Autodesk Fusion 360 part; units mm, degrees
(part 5 of 5)
component "TSSOP16_001" placed x (1, 0, 0) y (0, -1, 0) z (0, 0, -1) at (20.815, 10.6871, 0.1) in component "TSSOP16_010"
component "TSSOP16_002" placed x (1, 0, 0) y (0, -1, 0) z (0, 0, -1) at (20.815, 10.6871, 0.1) in component "TSSOP16_010"
component "TSSOP16_003" placed x (1, 0, 0) y (0, -1, 0) z (0, 0, -1) at (20.815, 10.6871, 0.1) in component "TSSOP16_010"
component "TSSOP16_004" placed x (1, 0, 0) y (0, -1, 0) z (0, 0, -1) at (20.815, 10.6871, 0.1) in component "TSSOP16_010"
component "TSSOP16_005" placed x (1, 0, 0) y (0, -1, 0) z (0, 0, -1) at (20.815, 10.6871, 0.1) in component "TSSOP16_010"
component "TSSOP16_006" placed x (1, 0, 0) y (0, -1, 0) z (0, 0, -1) at (20.815, 10.6871, 0.1) in component "TSSOP16_010"
component "TSSOP16_007" placed x (1, 0, 0) y (0, -1, 0) z (0, 0, -1) at (20.815, 10.6871, 0.1) in component "TSSOP16_010"
component "TSSOP16_008" placed x (1, 0, 0) y (0, -1, 0) z (0, 0, -1) at (20.815, 10.6871, 0.1) in component "TSSOP16_010"
component "TSSOP16_009" placed x (1, 0, 0) y (0, -1, 0) z (0, 0, -1) at (20.815, 10.6871, 0.1) in component "TSSOP16_010"
component "ShapeString253" placed x (1, 0, 0) y (0, 1, 0) z (0, 0, 1) at (0, 0, 0) in component "TSSOP16_010"
component "ShapeString001" placed x (1, 0, 0) y (0, 1, 0) z (0, 0, 1) at (-3.2, -0.84, 0) in component "ShapeString256"
component "ShapeString254" placed x (1, 0, 0) y (0, 1, 0) z (0, 0, 1) at (-3.2, -0.84, 0) in component "ShapeString256"
component "ShapeString255" placed x (1, 0, 0) y (0, 1, 0) z (0, 0, 1) at (-3.2, -0.84, 0) in component "ShapeString256"
component "ShapeString256" placed x (1, 0, 0) y (0, 1, 0) z (0, 0, 1) at (0, 0, 0) in component "Part010"
component "body" placed x (1, 0, 0) y (0, 1, 0) z (0, 0, 1) at (0, 0, 0) in component "SMD_resistor001"
component "contact1" placed x (1, 0, 0) y (0, 1, 0) z (0, 0, 1) at (0, -0.8, 0) in component "SMD_resistor001"
component "contact2" placed x (-1, 0, 0) y (0, -1, 0) z (0, 0, 1) at (0, 0.8, 0) in component "SMD_resistor001"
component "label" placed x (1, 0, 0) y (0, 1, 0) z (0, 0, 1) at (0, 0, 0.2) in component "SMD_resistor001"
component "Part010" placed x (0, 1, 0) y (-1, 0, 0) z (0, 0, 1) at (-0.66, 2.73, 0.24) in component "SMD_resistor001"
component "ShapeString002" placed x (1, 0, 0) y (0, 1, 0) z (0, 0, 1) at (-3.2, -0.84, 0) in component "ShapeString259"
component "ShapeString257" placed x (1, 0, 0) y (0, 1, 0) z (0, 0, 1) at (-3.2, -0.84, 0) in component "ShapeString259"
component "ShapeString258" placed x (1, 0, 0) y (0, 1, 0) z (0, 0, 1) at (-3.2, -0.84, 0) in component "ShapeString259"
component "ShapeString259" placed x (1, 0, 0) y (0, 1, 0) z (0, 0, 1) at (0, 0, 0) in component "Part013"
component "body003" placed x (1, 0, 0) y (0, 1, 0) z (0, 0, 1) at (0, 0, 0) in component "SMD_resistor002"
component "contact016" placed x (1, 0, 0) y (0, 1, 0) z (0, 0, 1) at (0, -0.8, 0) in component "SMD_resistor002"
component "contact017" placed x (-1, 0, 0) y (0, -1, 0) z (0, 0, 1) at (0, 0.8, 0) in component "SMD_resistor002"
component "label001" placed x (1, 0, 0) y (0, 1, 0) z (0, 0, 1) at (0, 0, 0.2) in component "SMD_resistor002"
component "Part013" placed x (0, 1, 0) y (-1, 0, 0) z (0, 0, 1) at (-0.66, 2.73, 0.24) in component "SMD_resistor002"
component "ShapeString003" placed x (1, 0, 0) y (0, 1, 0) z (0, 0, 1) at (-3.2, -0.84, 0) in component "ShapeString262"
component "ShapeString260" placed x (1, 0, 0) y (0, 1, 0) z (0, 0, 1) at (-3.2, -0.84, 0) in component "ShapeString262"
component "ShapeString261" placed x (1, 0, 0) y (0, 1, 0) z (0, 0, 1) at (-3.2, -0.84, 0) in component "ShapeString262"
component "ShapeString262" placed x (1, 0, 0) y (0, 1, 0) z (0, 0, 1) at (0, 0, 0) in component "Part015"
component "body004" placed x (1, 0, 0) y (0, 1, 0) z (0, 0, 1) at (0, 0, 0) in component "SMD_resistor003"
component "contact018" placed x (1, 0, 0) y (0, 1, 0) z (0, 0, 1) at (0, -0.8, 0) in component "SMD_resistor003"
component "contact019" placed x (-1, 0, 0) y (0, -1, 0) z (0, 0, 1) at (0, 0.8, 0) in component "SMD_resistor003"
component "label002" placed x (1, 0, 0) y (0, 1, 0) z (0, 0, 1) at (0, 0, 0.2) in component "SMD_resistor003"
component "Part015" placed x (0, 1, 0) y (-1, 0, 0) z (0, 0, 1) at (-0.66, 2.73, 0.24) in component "SMD_resistor003"
component "ShapeString004" placed x (1, 0, 0) y (0, 1, 0) z (0, 0, 1) at (-3.2, -0.84, 0) in component "ShapeString265"
component "ShapeString263" placed x (1, 0, 0) y (0, 1, 0) z (0, 0, 1) at (-3.2, -0.84, 0) in component "ShapeString265"
component "ShapeString264" placed x (1, 0, 0) y (0, 1, 0) z (0, 0, 1) at (-3.2, -0.84, 0) in component "ShapeString265"
component "ShapeString265" placed x (1, 0, 0) y (0, 1, 0) z (0, 0, 1) at (0, 0, 0) in component "Part017"
component "body005" placed x (1, 0, 0) y (0, 1, 0) z (0, 0, 1) at (0, 0, 0) in component "SMD_resistor004"
component "contact020" placed x (1, 0, 0) y (0, 1, 0) z (0, 0, 1) at (0, -0.8, 0) in component "SMD_resistor004"
component "contact021" placed x (-1, 0, 0) y (0, -1, 0) z (0, 0, 1) at (0, 0.8, 0) in component "SMD_resistor004"
component "label003" placed x (1, 0, 0) y (0, 1, 0) z (0, 0, 1) at (0, 0, 0.2) in component "SMD_resistor004"
component "Part017" placed x (0, 1, 0) y (-1, 0, 0) z (0, 0, 1) at (-0.66, 2.73, 0.24) in component "SMD_resistor004"
component "ShapeString005" placed x (1, 0, 0) y (0, 1, 0) z (0, 0, 1) at (-3.2, -0.84, 0) in component "ShapeString268"
component "ShapeString266" placed x (1, 0, 0) y (0, 1, 0) z (0, 0, 1) at (-3.2, -0.84, 0) in component "ShapeString268"
component "ShapeString267" placed x (1, 0, 0) y (0, 1, 0) z (0, 0, 1) at (-3.2, -0.84, 0) in component "ShapeString268"
component "ShapeString268" placed x (1, 0, 0) y (0, 1, 0) z (0, 0, 1) at (0, 0, 0) in component "Part019"
component "body006" placed x (1, 0, 0) y (0, 1, 0) z (0, 0, 1) at (0, 0, 0) in component "SMD_resistor005"
component "contact022" placed x (1, 0, 0) y (0, 1, 0) z (0, 0, 1) at (0, -0.8, 0) in component "SMD_resistor005"
component "contact023" placed x (-1, 0, 0) y (0, -1, 0) z (0, 0, 1) at (0, 0.8, 0) in component "SMD_resistor005"
component "label004" placed x (1, 0, 0) y (0, 1, 0) z (0, 0, 1) at (0, 0, 0.2) in component "SMD_resistor005"
component "Part019" placed x (0, 1, 0) y (-1, 0, 0) z (0, 0, 1) at (-0.66, 2.73, 0.24) in component "SMD_resistor005"
component "ShapeString006" placed x (1, 0, 0) y (0, 1, 0) z (0, 0, 1) at (-3.2, -0.84, 0) in component "ShapeString271"
component "ShapeString269" placed x (1, 0, 0) y (0, 1, 0) z (0, 0, 1) at (-3.2, -0.84, 0) in component "ShapeString271"
component "ShapeString270" placed x (1, 0, 0) y (0, 1, 0) z (0, 0, 1) at (-3.2, -0.84, 0) in component "ShapeString271"
component "ShapeString271" placed x (1, 0, 0) y (0, 1, 0) z (0, 0, 1) at (0, 0, 0) in component "Part021"
component "body007" placed x (1, 0, 0) y (0, 1, 0) z (0, 0, 1) at (0, 0, 0) in component "SMD_resistor006"
component "contact024" placed x (1, 0, 0) y (0, 1, 0) z (0, 0, 1) at (0, -0.8, 0) in component "SMD_resistor006"
component "contact025" placed x (-1, 0, 0) y (0, -1, 0) z (0, 0, 1) at (0, 0.8, 0) in component "SMD_resistor006"
component "label005" placed x (1, 0, 0) y (0, 1, 0) z (0, 0, 1) at (0, 0, 0.2) in component "SMD_resistor006"
component "Part021" placed x (0, 1, 0) y (-1, 0, 0) z (0, 0, 1) at (-0.66, 2.73, 0.24) in component "SMD_resistor006"
component "body008" placed x (1, 0, 0) y (0, 1, 0) z (0, 0, 1) at (0, 0, -0.015) in component "SMD_cap001"
component "contact026" placed x (1, 0, 0) y (0, 1, 0) z (0, 0, 1) at (0, 0.95, 0) in component "SMD_cap001"
component "contact027" placed x (-1, 0, 0) y (0, -1, 0) z (0, 0, 1) at (0, -0.94, 0) in component "SMD_cap001"
component "body002" placed x (1, 0, 0) y (0, 1, 0) z (0, 0, 1) at (0, 0, -0.015) in component "SMD_cap002"
component "contact014" placed x (1, 0, 0) y (0, 1, 0) z (0, 0, 1) at (0, 0.95, 0) in component "SMD_cap002"
component "contact015" placed x (-1, 0, 0) y (0, -1, 0) z (0, 0, 1) at (0, -0.94, 0) in component "SMD_cap002"
component "ShapeString064" placed x (1, 0, 0) y (0, 1, 0) z (0, 0, 1) at (-0.88, -0.26, 0.72) in component "ShapeString274"
component "ShapeString272" placed x (1, 0, 0) y (0, 1, 0) z (0, 0, 1) at (-0.88, -0.26, 0.72) in component "ShapeString274"
component "ShapeString273" placed x (1, 0, 0) y (0, 1, 0) z (0, 0, 1) at (-0.88, -0.26, 0.72) in component "ShapeString274"
component "ShapeString274" placed x (1, 0, 0) y (0, 1, 0) z (0, 0, 1) at (0, 0, 0) in component "SOT23"
component "Pin036" placed x (-1, 0, 0) y (0, -1, 0) z (0, 0, 1) at (0.905, -0.235, 0) in component "SOT23"
component "Pin035" placed x (-1, 0, 0) y (0, -1, 0) z (0, 0, 1) at (-0.965, -0.215, 0) in component "SOT23"
component "Pin1" placed x (1, 0, 0) y (0, 1, 0) z (0, 0, 1) at (0, 0.295, 0) in component "SOT23"
component "Case" placed x (1, 0, 0) y (0, 1, 0) z (0, 0, 1) at (0, 0, 0) in component "SOT23"
component "ShapeString065" placed x (1, 0, 0) y (0, 1, 0) z (0, 0, 1) at (-0.98, -0.36, 0.72) in component "ShapeString278"
component "ShapeString275" placed x (1, 0, 0) y (0, 1, 0) z (0, 0, 1) at (-0.98, -0.36, 0.72) in component "ShapeString278"
component "ShapeString276" placed x (1, 0, 0) y (0, 1, 0) z (0, 0, 1) at (-0.98, -0.36, 0.72) in component "ShapeString278"
component "ShapeString277" placed x (1, 0, 0) y (0, 1, 0) z (0, 0, 1) at (-0.98, -0.36, 0.72) in component "ShapeString278"
component "ShapeString278" placed x (1, 0, 0) y (0, 1, 0) z (0, 0, 1) at (0, 0, 0) in component "SOT23-1"
component "Pin039" placed x (-1, 0, 0) y (0, -1, 0) z (0, 0, 1) at (0.905, -0.235, 0) in component "SOT23-1"
component "Pin038" placed x (-1, 0, 0) y (0, -1, 0) z (0, 0, 1) at (-0.965, -0.215, 0) in component "SOT23-1"
component "Pin037" placed x (1, 0, 0) y (0, 1, 0) z (0, 0, 1) at (0, 0.295, 0) in component "SOT23-1"
component "Case001" placed x (1, 0, 0) y (0, 1, 0) z (0, 0, 1) at (0, 0, 0) in component "SOT23-1"
component "TSSOP16_010" placed x (0, -1, 0) y (1, 0, 0) z (0, 0, 1) at (-0.13, 1.12, -1.67) in component "parts"
component "SMD_resistor001" placed x (0, -1, 0) y (-1, 0, 0) z (0, 0, -1) at (-4.35, -27.4, -1.61) in component "parts"
component "SMD_resistor002" placed x (0, -1, 0) y (-1, 0, 0) z (0, 0, -1) at (-4.35, -20.25, -1.61) in component "parts"
component "SMD_resistor003" placed x (0, -1, 0) y (-1, 0, 0) z (0, 0, -1) at (13.1, -26.91, -1.61) in component "parts"
component "SMD_resistor004" placed x (0, -1, 0) y (-1, 0, 0) z (0, 0, -1) at (2.65, 0.38, -1.61) in component "parts"
component "SMD_resistor005" placed x (0, -1, 0) y (-1, 0, 0) z (0, 0, -1) at (2.65, 2.72, -1.61) in component "parts"
component "SMD_resistor006" placed x (0, -1, 0) y (-1, 0, 0) z (0, 0, -1) at (2.65, 4.99, -1.61) in component "parts"
component "SMD_cap001" placed x (0, -1, 0) y (1, 0, 0) z (0, 0, 1) at (13.15, -25.1, -2.1) in component "parts"
component "SMD_cap002" placed x (0, -1, 0) y (1, 0, 0) z (0, 0, 1) at (3, -20.2, -2.1) in component "parts"
component "SOT23" placed x (1, 0, 0) y (0, -1, 0) z (0, 0, -1) at (-4.1, -23.68, -2.02) in component "parts"
component "SOT23-1" placed x (0, -1, 0) y (-1, 0, 0) z (0, 0, -1) at (2.67, -24, -2.02) in component "parts"
component "Frame" placed x (1, 0, 0) y (0, 1, 0) z (0, 0, 1) at (0, 0, 2.5) in component "pls-14"
component "Pin01" placed x (1, 0, 0) y (0, 1, 0) z (0, 0, 1) at (-16.51, 0, 0) in component "pls-14"
component "Pin002" placed x (1, 0, 0) y (0, 1, 0) z (0, 0, 1) at (-13.97, 0, 0) in component "pls-14"
component "Pin003" placed x (1, 0, 0) y (0, 1, 0) z (0, 0, 1) at (-11.43, 0, 0) in component "pls-14"
component "Pin004" placed x (1, 0, 0) y (0, 1, 0) z (0, 0, 1) at (-8.89, 0, 0) in component "pls-14"
component "Pin005" placed x (1, 0, 0) y (0, 1, 0) z (0, 0, 1) at (-6.35, 0, 0) in component "pls-14"
component "Pin006" placed x (1, 0, 0) y (0, 1, 0) z (0, 0, 1) at (-3.81, 0, 0) in component "pls-14"
component "Pin007" placed x (1, 0, 0) y (0, 1, 0) z (0, 0, 1) at (-1.27, 0, 0) in component "pls-14"
component "Pin008" placed x (1, 0, 0) y (0, 1, 0) z (0, 0, 1) at (1.27, 0, 0) in component "pls-14"
component "Pin009" placed x (1, 0, 0) y (0, 1, 0) z (0, 0, 1) at (3.81, 0, 0) in component "pls-14"
component "Pin010" placed x (1, 0, 0) y (0, 1, 0) z (0, 0, 1) at (6.35, 0, 0) in component "pls-14"
component "Pin011" placed x (1, 0, 0) y (0, 1, 0) z (0, 0, 1) at (8.89, 0, 0) in component "pls-14"
component "Pin012" placed x (1, 0, 0) y (0, 1, 0) z (0, 0, 1) at (11.43, 0, 0) in component "pls-14"
component "Pin013" placed x (1, 0, 0) y (0, 1, 0) z (0, 0, 1) at (13.97, 0, 0) in component "pls-14"
component "Pin014" placed x (1, 0, 0) y (0, 1, 0) z (0, 0, 1) at (16.51, 0, 0) in component "pls-14"
component "SD slot" placed x (0, 1, 0) y (1, 0, 0) z (0, 0, -1) at (-16.32, 3.6, -0.3) in component "components"
component "parts" placed x (1, 0, 0) y (0, 1, 0) z (0, 0, 1) at (0, 0, 1.31) in component "components"
component "pls-14" placed x (-1, 0, 0) y (0, 1, 0) z (0, 0, -1) at (0, -41, 2.28) in component "components"
component "plate and holes" placed x (1, 0, 0) y (0, 1, 0) z (0, 0, 1) at (0, 0, 0) in component "Board"
component "silk_upper" placed x (1, 0, 0) y (0, 1, 0) z (0, 0, 1) at (0, 0, 1.82) in component "Board"
component "cupper_upper" placed x (1, 0, 0) y (0, 1, 0) z (0, 0, 1) at (0, 0, 1.6) in component "Board"
component "cupper_bottom" placed x (1, 0, 0) y (0, 1, 0) z (0, 0, 1) at (0, 0, -0.1) in component "Board"
component "mask_bottom" placed x (1, 0, 0) y (0, 1, 0) z (0, 0, 1) at (0, 0, -0.2) in component "Board"
component "silk_bottom" placed x (1, 0, 0) y (0, 1, 0) z (0, 0, 1) at (0, 0, -0.01) in component "Board"
component "components" placed x (1, 0, 0) y (0, 1, 0) z (0, 0, 1) at (0, 0, 0) in component "Board"
component "mask_upper" placed x (1, 0, 0) y (0, 1, 0) z (0, 0, 1) at (0, 0, 1.7) in component "Board"
component "light_shelf" placed x (1, 0, 0) y (0, 0, -1) z (0, 1, 0) at (0, -30.43, -30.75) in component "tft_cable"
component "main_shelf" placed x (1, 0, 0) y (0, 1, 0) z (0, 0, 1) at (0, 0, 0) in component "tft_cable"
component "tft_cable" placed x (1, 0, 0) y (0, -1, 0) z (0, 0, -1) at (-12.5, -65.5, -0.43) in component "tft"
component "tft_matrix" placed x (1, 0, 0) y (0, 1, 0) z (0, 0, 1) at (0, 2.96, 1.5) in component "tft"
component "tft_board" placed x (1, 0, 0) y (0, 1, 0) z (0, 0, 1) at (0, 0, 0) in component "tft"
component "screen_film" placed x (1, 0, 0) y (0, 1, 0) z (0, 0, 1) at (0, 0, 0) in component "screen"
component "screen_glass" placed x (1, 0, 0) y (0, 1, 0) z (0, 0, 1) at (0, 0, 0.22) in component "screen"
component "frame" placed x (1, 0, 0) y (0, 1, 0) z (0, 0, 1) at (0, 2, 0.23) in component "Display"
component "metal bandage" placed x (1, 0, 0) y (0, 1, 0) z (0, 0, 1) at (0, 0, 0) in component "Display"
component "tft" placed x (1, 0, 0) y (0, 1, 0) z (0, 0, 1) at (0, 2.3, 0.65) in component "Display"
component "screen" placed x (1, 0, 0) y (0, 1, 0) z (0, 0, 1) at (0, 2, 2.65) in component "Display"
component "ShapeString068" placed x (0, 1, 0) y (1, 0, 0) z (0, 0, -1) at (16.1, -39.5, 0) in component "touch_cable"
component "touch_cable_contacts" placed x (1, 0, 0) y (0, 1, 0) z (0, 0, 1) at (0, 0, 0) in component "touch_cable"
component "touch_cable_film" placed x (1, 0, 0) y (0, 1, 0) z (0, 0, 1) at (0, 0, 0.1) in component "touch_cable"
component "touch_routs" placed x (1, 0, 0) y (0, 1, 0) z (0, 0, 1) at (0, 0, 0.05) in component "Touchscreen"
component "touch_protect" placed x (1, 0, 0) y (0, 1, 0) z (0, 0, 1) at (0, 0, 0.15) in component "Touchscreen"
component "touch_cable" placed x (1, 0, 0) y (0, 1, 0) z (0, 0, 1) at (-12.6, -4, 3.7) in component "Touchscreen"
component "Display" placed x (1, 0, 0) y (0, 1, 0) z (0, 0, 1) at (0, 0, 0) in component "Display and Touchscreen"
component "Touchscreen" placed x (1, 0, 0) y (0, 1, 0) z (0, 0, 1) at (0, 0, 0) in component "Display and Touchscreen"
component "Board" placed x (1, 0, 0) y (0, 1, 0) z (0, 0, 1) at (0, 0, 0) in component "2.8''LCD_MSP2807"
component "Display and Touchscreen" placed x (1, 0, 0) y (0, 1, 0) z (0, 0, 1) at (0, 0, 1.89) in component "2.8''LCD_MSP2807"
component "2.8''LCD_MSP2807" placed x (1, 0, 0) y (0, 1, 0) z (0, 0, 1) at (0, 0, 0) in component "LCD_MSP2807_fusion"
component "VS-1213-67-160GF" placed x (1, 0, 0) y (0, 1, 0) z (0, 0, 1) at (0, 0, 0) in component "VS-1213-67-160GF (1)"
component "C_1206_3216Metric" placed x (1, 0, 0) y (0, 1, 0) z (0, 0, 1) at (0, 0, 0) in component "C_1206_3216Metric (1)"
component "TF-SMD_TF-012" placed x (1, 0, 0) y (0, 1, 0) z (0, 0, 1) at (0, 0, 0) in component "TF-SMD_TF-012 (1)"
component "ESP32 S3 SUPERMINI" placed x (1, 0, 0) y (0, 1, 0) z (0, 0, 1) at (0, 0, 0) in component "ESP32-S3-ZERO"
component "FCR684205R ORJ5" placed x (1, 0, 0) y (0, 1, 0) z (0, 0, 1) at (0, 0, 0) in component "4654_FCR684205T%20OTJ5"
